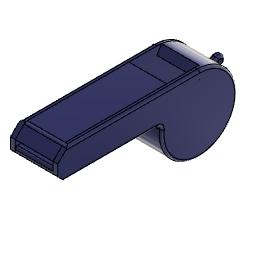
whistle v1 (Autodesk Fusion 360 design; units mm, degrees)
Autodesk Fusion 360 part; units mm, degrees
note: some values were not read from the file. Chosen so that the rebuilt part matches the saved one: which face or edge a step refers to; which pieces of a blend or face edit are solid.
sketch "Sketch1" plane through (0, 0, 0) normal (1, 0, 0) x (0, 1, 0)
  line L0 (44, 0) -> (60, 0)
  line L1 (48.157281, 16) -> (0, 16)
  line L2 (0, 11) -> (48.157281, 11)
  line L3 (0, 4) -> (48.157281, 4)
  line L4 (60, 12.5) -> (61.95174, 15.880514)
  line L5 (0, 9) -> (48.157281, 9)
  arc A0 (48.157281, 4) -> (60, 12.5) centre (60, 0) ccw
  arc A1 (44.508067, 4) -> (61.95174, 15.880514) centre (60, 0) ccw
  line L6 (48.157281, 4) -> (48.157281, 9)
  line L7 (48.157281, 11) -> (48.157281, 16)
  line L8 (0, 16) -> (0, 11)
  line L9 (0, 9) -> (0, 4)
  circle A2 centre (77.535082, 6.382248) radius 1
  arc A3 (73.515624, 8.563171) -> (76.37008, 8.007908) centre (75.205077, 9.633567) ccw
  arc A4 (77.687592, 4.388071) -> (75.857869, 2.127906) centre (77.840103, 2.393895) ccw
  arc A5 (77.687592, 4.388071) -> (76.37008, 8.007908) centre (77.535082, 6.382248) ccw
  point P0 (75.035082, 5.472322)
  dimension "d1" = 60
  dimension "d3" = 25
  dimension "d8" = 5
  dimension "d10" = 12
  dimension "d13" = 7
  dimension "d16" = 4
  dimension "d17" = 2
  dimension "d18" = 2.5
  dimension "d19" = 4
  dimension "d20" = 4
  constraint horizontal L0
  constraint parallel L0 L1
  constraint perpendicular L0 L8
  constraint perpendicular L2 L8
  constraint perpendicular L5 L8
  constraint perpendicular L3 L8
  constraint perpendicular L1 L6
  constraint collinear L6 L7
  constraint collinear L8 L9
  constraint concentric A2 A5
  constraint tangent A4 A5
  constraint tangent A1 A4
  constraint tangent A3 A5
  constraint tangent A1 A3
  measures "d1" distance of origin L0.end
  measures "d3" diameter of A0
  measures "d8" distance of L1 L2
  measures "d10" distance of L1 L3
  measures "d13" distance of L1 L5
  measures "d16" diameter of A5
  measures "d17" diameter of A2
  measures "d19" diameter of A3
  measures "d20" diameter of A4
sketch "Sketch2" plane through (0, 0, 0) normal (1, 0, 0) x (0, 1, 0)
sketch "Sketch3" plane through (0, 0, 0) normal (1, 0, 0) x (0, 1, 0)
extrude "Extrude1" add sketch "Sketch1" along normal blind 8 and the other way blind 8 contours L0 L3 A0 A1 | L0 L4 A0 A1 | L3 L5 L6 L9 | L1 L2 L7 L8 picked at (46.531216, 2.243399) picked at (74.765254, 1.035185) picked at (30.888449, 7.333333) picked at (16.052427, 14.333333) makes body 1 at (2.666667, 71.001955, 11.617099) makes body 2 at (-2.666667, 16.052427, 11)
extrude "Extrude2" add sketch "Sketch1" along normal blind 1.5 and the other way blind 1.5 contours A1 A3 A4 A5 picked at (75.523999, 5.667955) bodies 1
sketch "Sketch4" plane through (8, 0, 0) normal (1, 0, 0) x (0, 1, 0)
  line L0 (48.157281, 4) -> (48.157281, 9)
  line L1 (48.157281, 9) -> (0, 9)
  line L2 (0, 9) -> (0, 4)
  line L3 (0, 4) -> (44.508067, 4)
  arc A0 (44.508067, 4) -> (61.95174, 15.880514) centre (60, 0) ccw
  line L4 (61.95174, 15.880514) -> (60, 12.5)
  arc A1 (48.157281, 4) -> (60, 12.5) centre (60, 0) ccw
  line L5 (0, 4) -> (48.157281, 4)
  line L6 (60.053107, 12.499887) -> (60.053107, 12.591983)
  line L7 (60.053107, 15.999912) -> (0, 15.999912)
  line L8 (0, 15.999912) -> (0, 4)
  arc A2 (44.508067, 4) -> (59.946893, 15.999912) centre (60, 0) ccw
  dimension "d29" = 32
  constraint concentric A0 A2
  constraint horizontal L5
  constraint vertical L6
  constraint horizontal L7
  constraint vertical L8
  constraint coincident L2.end L3.start
  measures "d29" diameter of A2
extrude "Extrude3" add sketch "Sketch4" along normal blind 2 contours L0 L1 L2 L3 L5 L8 | L0 L1 L4 A1 L7 L8 A2 | A0 L4 A1 L5 L6 A2 picked at (30.888449, 7.333333) picked at (59.696521, 3.47968) picked at (45.431511, 2.633655) bodies 2 1
sketch "Sketch5" plane through (-8, 0, 0) normal (-1, 0, 0) x (0, -1, 0)
  line L0 (-48.157281, 9) -> (-48.157281, 4)
  arc A0 (-60, 12.5) -> (-48.157281, 4) centre (-60, 0) ccw
  line L1 (-60, 12.5) -> (-61.95174, 15.880514)
  arc A1 (-61.95174, 15.880514) -> (-44.508067, 4) centre (-60, 0) ccw
  line L2 (-44.508067, 4) -> (0, 4)
  line L3 (0, 4) -> (0, 9)
  line L4 (0, 9) -> (-48.157281, 9)
  line L5 (0, 4) -> (-44.508067, 4)
  line L6 (-60, 16) -> (0, 16)
  line L7 (0, 16) -> (0, 4)
  arc A2 (-60, 16) -> (-44.508067, 4) centre (-60, 0) ccw
  dimension "d32" = 32
  constraint concentric A0 A2
  constraint horizontal L5
  constraint horizontal L6
  constraint vertical L7
  constraint coincident L2.end L3.start
  measures "d32" diameter of A2
extrude "Extrude4" add sketch "Sketch5" along normal blind 2 separate body contours L0 A0 L1 A1 L2 L3 L4 L5 L7 A2 | L0 A0 L1 L4 L6 L7 A2 picked at (-30.888449, 7.333333) picked at (-36.052427, 13.666667) makes body 3
chamfer "Chamfer1" distance 4.355 distance2 4.355 3 edges at (-9, 0, 16) (0, 0, 16) (9, 0, 15.999912) measured on face at (-8.666667, 0, 13.666667) measured on face at (3.333333, 0, 5.666667) measured on face at (9.333333, 36.070129, 15.999912) on bodies 2 3
chamfer "Chamfer2" distance 3 distance2 3 1 edges at (-9, 0, 4) measured on face at (-8.666667, 29.672044, 4) on bodies 3
chamfer "Chamfer3" distance 3 distance2 3 1 edges at (1, 0, 4) measured on face at (3.333333, 0, 5.666667) on bodies 2
fillet "Fillet1" radius 2 4 edges at (9, 4.354912, 15.999912) (8, 4.354956, 15.999956) (0, 4.355, 16) (1, 44.508067, 4) on bodies 2
fillet "Fillet2" radius 1 2 edges at (0, 0, 11) (0, 0, 9) on bodies 2
fillet "Fillet3" radius 1 6 edges at (1.5, 76.285635, 3.652318) (1.5, 79.414467, 7.066288) (1.5, 74.823185, 7.670366) (-1.5, 74.823185, 7.670366) (-1.5, 79.414467, 7.066288) (-1.5, 76.285635, 3.652318) on bodies 2
fillet "Fillet4" radius 1 2 edges at (-10, 32.1775, 16) (-10, 69.797959, -12.649111) on bodies 3
fillet "Fillet5" radius 1 1 edges at (-10, 24.271584, 4) on bodies 3
fillet "Fillet6" radius 1 4 edges at (10, 70.64686, -11.943382) (10, 43.602168, 3.333333) (10, 22.555728, 4) (10, 32.608879, 15.999912) on bodies 2
